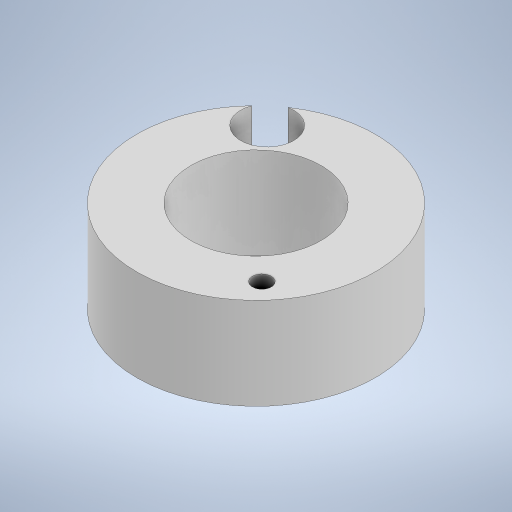
# Autodesk Inventor part: rhtgt; gjlibgybrf
Saved by Autodesk Inventor 2024.2 (Build 282272000, 272)
## iProperties
Created: 2026-03-15
Part Number: rhtgt; gjlibgybrf
Material: Типовые
Document SubType Name: Modeling
Designer: Service
Density: 1 g/cm^3
Appearance: По умолчанию
Author: Service
Autodesk Inventor part; units mm, degrees
ref_plane "YZ Plane" through (0, 0, 0) normal (1, 0, 0) x (0, 1, 0)
ref_plane "XZ Plane" through (0, 0, 0) normal (0, 1, 0) x (-1, 0, 0)
ref_plane "XY Plane" through (0, 0, 0) normal (0, 0, 1) x (1, 0, 0)
sketch "Эскиз1" plane through (0, 0, 0) normal (0, 1, 0) x (-1, 0, 0)
  circle A0 centre (0, 0) radius 13
  circle A1 centre (0, 0) radius 7.1
  circle A2 centre (-7.739, 7.1) radius 1.0298
  circle A3 centre (6.719, -7.9386) radius 2.8878
  point P0 (7.278, -10.7718)
  point P1 (9.4208, -8.9581)
  dimension "d0" = 26
  dimension "d1" = 14.2
  constraints: 4 centre point, 2 coincident
  measures "d0" diameter of A0
  measures "d1" diameter of A1
extrude "Выдавливание1" add sketch "Эскиз1" along normal blind 10 contours A0 A3 picked at (-9.201, 3.672)
